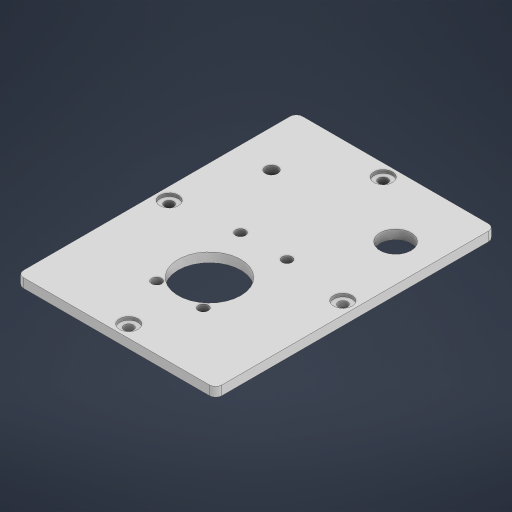
# Autodesk Inventor part: Case Top
Saved by Autodesk Inventor 2024 (Build 280153000, 153)
## iProperties
Created: 2023-06-21
Part Number: Case Top
Material: Generic
Document SubType Name: Modeling
Designer: Aryasetya
Density: 1 g/cm^3
Appearance: Default
Author: Aryasetya
Autodesk Inventor part; units mm, degrees
ref_plane "YZ Plane" through (0, 0, 0) normal (1, 0, 0) x (0, 1, 0)
ref_plane "XZ Plane" through (0, 0, 0) normal (0, 1, 0) x (-1, 0, 0)
ref_plane "XY Plane" through (0, 0, 0) normal (0, 0, 1) x (1, 0, 0)
sketch "Sketch1" plane through (0, 0, 0) normal (0, 1, 0) x (-1, 0, 0)
  line L0 (-30, -43) -> (30, -43)
  line L1 (30, -43) -> (30, 43)
  line L2 (30, 43) -> (-30, 43)
  line L3 (-30, 43) -> (-30, -43)
  line L4 (-30, -43) -> (30, 43) construction
  line L5 (30, -43) -> (-30, 43) construction
  line L6 (0, 43) -> (0, 45)
  line L7 (30, 0) -> (32, 0)
  line L8 (-30, -45) -> (30, -45)
  line L9 (32, -43) -> (32, 43)
  line L10 (30, 45) -> (-30, 45)
  line L11 (-32, 43) -> (-32, -43)
  line L12 (-32, -45) -> (32, 45) construction
  line L13 (32, -45) -> (-32, 45) construction
  arc A0 (-32, -43) -> (-30, -45) centre (-30, -43) ccw
  arc A1 (30, -45) -> (32, -43) centre (30, -43) ccw
  arc A2 (32, 43) -> (30, 45) centre (30, 43) ccw
  arc A3 (-30, 45) -> (-32, 43) centre (-30, 43) ccw
  point P0 (0, 0)
  point P1 (0, 0)
  dimension "d4" = 60
  dimension "d5" = 86
  dimension "d6" = 2
  dimension "d7" = 2
  dimension "d8" = 2
  constraints: 28 end point, 8 point on circle, 8 point on line, 8 tangent, 6 midpoint, 4 centre point, 4 parallel, 3 equal radius, 3 horizontal, 2 perpendicular, 1 vertical
  measures "d4" distance of L3.start L1.end
  measures "d5" distance of L1.end L1.start
  measures "d6" distance of L6.start L6.end
  measures "d7" distance of L7.start L7.end
  measures "d8" radius of A0
extrude "Extrusion1" add sketch "Sketch1" along normal blind 3
sketch "Sketch2" plane through (0, 3, 0) normal (0, 1, 0) x (1, 0, 0)
  circle A0 centre (0, 41) radius 1.5
  circle A1 centre (-28, 0) radius 1.5
  circle A2 centre (0, -41) radius 1.5
  circle A3 centre (28, 0) radius 1.5
  line L0 (-32, 43) -> (-32, -43)
  arc A4 (-32, -43) -> (-30, -45) centre (-30, -43) ccw
  line L1 (-30, -45) -> (30, -45)
  arc A5 (-30, 45) -> (-32, 43) centre (-30, 43) ccw
  line L2 (30, 45) -> (-30, 45)
  arc A6 (32, 43) -> (30, 45) centre (30, 43) ccw
  line L3 (32, -43) -> (32, 43)
  arc A7 (30, -45) -> (32, -43) centre (30, -43) ccw
  circle A8 centre (-20, 25) radius 2
  circle A9 centre (7.5, 2.5) radius 1.6
  circle A10 centre (7.5, -24.5) radius 1.6
  circle A11 centre (0, -15) radius 10.1
  circle A12 centre (-7.5, 2.5) radius 1.6
  circle A13 centre (-7.5, -24.5) radius 1.6
  line L4 (0, 0) -> (0, 4.1)
  circle A14 centre (20, 25) radius 5
  point P0 (-5.5, -13.5)
  dimension "d11" = 4
  dimension "d13" = 20.2
  dimension "d14" = 3.2
  dimension "d15" = 3.2
  dimension "d16" = 3.2
  dimension "d17" = 3.2
  dimension "d20" = 10
  constraints: 15 centre point, 10 end point, 8 point on circle, 1 vertical
  measures "d11" diameter of A8
  measures "d13" diameter of A11
  measures "d14" diameter of A13
  measures "d15" diameter of A10
  measures "d16" diameter of A12
  measures "d17" diameter of A9
  measures "d20" diameter of A14
extrude "Extrusion2" cut sketch "Sketch2" against normal through all contours A0 | A1 | A2 | A3 | A8 | A9 | A10 | A11 | A12 | A13 | A14
sketch "Sketch3" plane through (0, 3, 0) normal (0, 1, 0) x (1, 0, 0)
  circle A0 centre (-28, 0) radius 1.5 projected
  circle A1 centre (0, 41) radius 1.5 projected
  circle A2 centre (0, -41) radius 1.5 projected
  circle A3 centre (28, 0) radius 1.5 projected
  circle A4 centre (0, -41) radius 3
  circle A5 centre (-28, 0) radius 3
  circle A6 centre (0, 41) radius 3
  circle A7 centre (28, 0) radius 3
  point P0 (0, 0)
  dimension "d21" = 6
  dimension "d22" = 6
  dimension "d23" = 6
  dimension "d24" = 6
  constraints: 4 centre point, 4 coincident
  measures "d21" diameter of A4
  measures "d22" diameter of A5
  measures "d23" diameter of A6
  measures "d24" diameter of A7
extrude "Extrusion3" cut sketch "Sketch3" against normal blind 1
body "Solid1"
